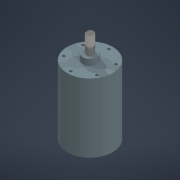
# Autodesk Inventor part: Motor24V_V1
Saved by Autodesk Inventor 2022.2 (Build 262287000, 287)
## iProperties
Created: 2022-11-20
Part Number: Motor24V_V1
Material: Steel
Document SubType Name: Modeling
Designer: jaege
Density: 7.85 g/cm^3
Appearance: Galvanized
Author: jaege
Autodesk Inventor part; units mm, degrees
ref_plane "YZ Plane" through (0, 0, 0) normal (1, 0, 0) x (0, 1, 0)
ref_plane "XZ Plane" through (0, 0, 0) normal (0, 1, 0) x (-1, 0, 0)
ref_plane "XY Plane" through (0, 0, 0) normal (0, 0, 1) x (1, 0, 0)
sketch "Sketch1" plane through (0, 0, 0) normal (0, 1, 0) x (-1, 0, 0)
  circle A0 centre (0, 0) radius 18.5
  dimension "d0" = 37
  constraints: 1 centre point, 1 coincident
  measures "d0" diameter of A0
extrude "Extrusion1" add sketch "Sketch1" along normal blind 55.8
sketch "Sketch2" plane through (0, 55.8, 0) normal (0, 1, 0) x (1, 0, 0)
  circle A0 centre (0, 0) radius 6
  dimension "d3" = 12
  constraints: 1 centre point, 1 coincident
  measures "d3" diameter of A0
extrude "Extrusion2" add sketch "Sketch2" along normal blind 5
sketch "Sketch3" plane through (0, 60.8, 0) normal (0, 1, 0) x (1, 0, 0)
  circle A0 centre (0, 0) radius 3
  line L0 (-2.5, -3) -> (3, -3)
  line L1 (3, -3) -> (3, 3)
  line L2 (3, 3) -> (-2.5, 3)
  line L3 (-2.5, 3) -> (-2.5, -3)
  point P0 (-2.5, 1.6583)
  point P1 (-2.5, -1.6583)
  dimension "d6" = 6
  dimension "d7" = 5.5
  constraints: 8 end point, 3 tangent, 2 parallel, 1 centre point, 1 coincident, 1 horizontal, 1 perpendicular
  measures "d6" diameter of A0
  measures "d7" distance of L1.end L2.end
extrude "Extrusion3" add sketch "Sketch3" along normal blind 14 contours A0 L3 picked at (0.6006, -0.3482)
sketch "Sketch4" plane through (0, 0, 0) normal (0, -1, 0) x (1, 0, 0)
  circle A0 centre (0, 0) radius 17.5
  circle A1 centre (0, 0) radius 18.5 projected
  dimension "d27" = 1
  constraints: 1 centre point, 1 coincident
  measures "d27" radial gap between concentric circles of A0 A1
extrude "Extrusion4" cut sketch "Sketch4" against normal blind 1 contours A0
sketch "Sketch5" plane through (0, 1, 0) normal (0, -1, 0) x (1, 0, 0)
  circle A0 centre (0, 0) radius 18.5 projected
  circle A1 centre (0, 0) radius 5
  dimension "d13" = 10
  constraints: 1 centre point, 1 coincident
  measures "d13" diameter of A1
extrude "Extrusion5" add sketch "Sketch5" along normal blind 2 contours A1
sketch "Sketch7" plane through (0, 55.8, 0) normal (0, 1, 0) x (1, 0, 0)
  line L0 (0, 25.9) -> (0, -25.9) projected
  point P0 (0, 0)
  point P1 (0, 15.5)
  point P2 (-13.4234, 7.75)
  point P3 (-13.4234, -7.75)
  point P4 (0, -15.5)
  point P5 (13.4234, -7.75)
  point P6 (13.4234, 7.75)
  dimension "d35" = 15.5
  dimension "d38" = 360
  constraints: 1 point on line, 7 other
  measures "d35" distance of point (0, 0) point (0, 15.5)
hole "Hole1" at (-13.4234, 55.8, -7.75) at (-13.4234, 55.8, 7.75) at (13.4234, 55.8, 7.75) at (13.4234, 55.8, -7.75) at (0, 55.8, -15.5) at (0, 55.8, 15.5) direction (0, -1, 0) diameter 2.459 depth 8.8 tip angle 118 thread size "M3x0.5" class "6H" standard "ANSI Metric M Profile"
sketch "Sketch8" plane through (0, 1, 0) normal (0, -1, 0) x (1, 0, 0)
  line L0 (-11.5, -1.5) -> (-11, -1.5)
  line L1 (-11, -1.5) -> (-11, 1.5)
  line L2 (-11, 1.5) -> (-11.5, 1.5)
  line L3 (-11.5, 1.5) -> (-11.5, -1.5)
  line L4 (11, -1.5) -> (11.5, -1.5)
  line L5 (11.5, -1.5) -> (11.5, 1.5)
  line L6 (11.5, 1.5) -> (11, 1.5)
  line L7 (11, 1.5) -> (11, -1.5)
  circle A0 centre (0, 0) radius 5 projected
  circle A1 centre (0, 0) radius 17.5 projected
  line L8 (0, -17.5) -> (0, 17.5) construction
  point P0 (-11, 0)
  point P1 (11, 0)
  dimension "d30" = 23
  dimension "d31" = 0.5
  dimension "d32" = 0.5
  dimension "d33" = 3
  dimension "d34" = 3
  constraints: 18 end point, 4 parallel, 2 horizontal, 2 horizontal alignment, 2 midpoint, 2 perpendicular, 2 point on circle, 1 vertical, 1 vertical alignment, 1 other
  measures "d30" distance between parallel lines of L3 L5
  measures "d31" distance of L0.start L0.end
  measures "d32" distance of L4.start L4.end
  measures "d33" distance of L4.end L5.end
  measures "d34" distance of L2.end L0.start
extrude "Extrusion7" add sketch "Sketch8" along normal blind 6.5 contours L3 L2 L1 L0 | L7 L6 L5 L4
body "Solid1"
